Autodesk Fusion 360 part; units mm, degrees
(part 2 of 7)
  spline S12 degree 5 poles (-1.6341, -11.6319) (-1.6348, -11.637) (-1.6361, -11.6471) (-1.6376, -11.6624) (-1.639, -11.6827) (-1.6398, -11.7083) (-1.6398, -11.7339) (-1.6394, -11.7596) (-1.6387, -11.7853) (-1.6379, -11.8111) (-1.6369, -11.8368) (-1.6357, -11.8626) (-1.6342, -11.8884) (-1.6324, -11.9143) (-1.6302, -11.9401) (-1.6277, -11.966) (-1.6249, -11.9919) (-1.6219, -12.0178) (-1.6187, -12.0438) (-1.6153, -12.0697) (-1.6117, -12.0957) (-1.608, -12.1216) (-1.604, -12.1476) (-1.5998, -12.1736) (-1.5953, -12.1996) (-1.5907, -12.2256) (-1.5859, -12.2517) (-1.5809, -12.2777) (-1.5757, -12.3037) (-1.5703, -12.3298) (-1.5648, -12.3558) (-1.5591, -12.3818) (-1.5532, -12.4079) (-1.5471, -12.4339) (-1.5409, -12.46) (-1.5345, -12.4861) (-1.5279, -12.5121) (-1.5212, -12.5382) (-1.5143, -12.5642) (-1.5072, -12.5903) (-1.5, -12.6164) (-1.4927, -12.6424) (-1.4851, -12.6685) (-1.4775, -12.6945) (-1.4696, -12.7206) (-1.4617, -12.7466) (-1.4535, -12.7727) (-1.4453, -12.7987) (-1.4368, -12.8247) (-1.4283, -12.8508) (-1.4196, -12.8768) (-1.4107, -12.9028) (-1.4017, -12.9288) (-1.3926, -12.9548) (-1.3833, -12.9808) (-1.3739, -13.0068) (-1.3643, -13.0328) (-1.3546, -13.0588) (-1.3448, -13.0848) (-1.3348, -13.1107) (-1.3247, -13.1367) (-1.3144, -13.1626) (-1.3041, -13.1885) (-1.2936, -13.2145) (-1.2829, -13.2404) (-1.2721, -13.2663) (-1.2612, -13.2921) (-1.2502, -13.318) (-1.239, -13.3439) (-1.2278, -13.3697) (-1.2163, -13.3956) (-1.2071, -13.4162) (-1.2001, -13.4317) (-1.1954, -13.442) (-1.1931, -13.4472) knots 0 0 0 0 0 0 0.01428571 0.02857143 0.04285714 0.05714286 0.07142857 0.08571429 0.1 0.11428571 0.12857143 0.14285714 0.15714286 0.17142857 0.18571429 0.2 0.21428571 0.22857143 0.24285714 0.25714286 0.27142857 0.28571429 0.3 0.31428571 0.32857143 0.34285714 0.35714286 0.37142857 0.38571429 0.4 0.41428571 0.42857143 0.44285714 0.45714286 0.47142857 0.48571429 0.5 0.51428571 0.52857143 0.54285714 0.55714286 0.57142857 0.58571429 0.6 0.61428571 0.62857143 0.64285714 0.65714286 0.67142857 0.68571429 0.7 0.71428571 0.72857143 0.74285714 0.75714286 0.77142857 0.78571429 0.8 0.81428571 0.82857143 0.84285714 0.85714286 0.87142857 0.88571429 0.9 0.91428571 0.92857143 0.94285714 0.95714286 0.97142857 0.98571429 1 1 1 1 1 1
  arc A26 (-1.1931, -13.4472) -> (-0.5017, -13.4907) centre (0, 0) ccw
  spline S13 degree 5 poles (-0.5017, -13.4907) (-0.4987, -13.4858) (-0.4928, -13.4762) (-0.4839, -13.4617) (-0.4722, -13.4424) (-0.4576, -13.4182) (-0.4432, -13.3939) (-0.4288, -13.3697) (-0.4147, -13.3454) (-0.4006, -13.3211) (-0.3867, -13.2967) (-0.3729, -13.2724) (-0.3592, -13.248) (-0.3456, -13.2236) (-0.3322, -13.1991) (-0.3189, -13.1746) (-0.3058, -13.1501) (-0.2928, -13.1256) (-0.2799, -13.101) (-0.2672, -13.0765) (-0.2546, -13.0519) (-0.2421, -13.0272) (-0.2298, -13.0026) (-0.2176, -12.9779) (-0.2055, -12.9532) (-0.1936, -12.9285) (-0.1819, -12.9037) (-0.1702, -12.8789) (-0.1588, -12.8541) (-0.1474, -12.8293) (-0.1363, -12.8045) (-0.1252, -12.7796) (-0.1143, -12.7547) (-0.1036, -12.7298) (-0.093, -12.7049) (-0.0826, -12.6799) (-0.0724, -12.655) (-0.0623, -12.63) (-0.0523, -12.605) (-0.0425, -12.5799) (-0.0329, -12.5549) (-0.0235, -12.5298) (-0.0142, -12.5047) (-0.0051, -12.4796) (0.0039, -12.4545) (0.0126, -12.4293) (0.0212, -12.4042) (0.0296, -12.379) (0.0378, -12.3538) (0.0459, -12.3286) (0.0537, -12.3034) (0.0614, -12.2781) (0.0688, -12.2529) (0.076, -12.2276) (0.083, -12.2023) (0.0899, -12.177) (0.0965, -12.1517) (0.1029, -12.1264) (0.1091, -12.101) (0.1151, -12.0757) (0.1209, -12.0503) (0.1263, -12.0249) (0.1313, -11.9995) (0.136, -11.9741) (0.1404, -11.9487) (0.1447, -11.9232) (0.1487, -11.8978) (0.1526, -11.8724) (0.1562, -11.8469) (0.1594, -11.8215) (0.1619, -11.796) (0.1631, -11.7757) (0.1634, -11.7603) (0.1634, -11.7501) (0.1633, -11.745) knots -1 -1 -1 -1 -1 -1 -0.98571429 -0.97142857 -0.95714286 -0.94285714 -0.92857143 -0.91428571 -0.9 -0.88571429 -0.87142857 -0.85714286 -0.84285714 -0.82857143 -0.81428571 -0.8 -0.78571429 -0.77142857 -0.75714286 -0.74285714 -0.72857143 -0.71428571 -0.7 -0.68571429 -0.67142857 -0.65714286 -0.64285714 -0.62857143 -0.61428571 -0.6 -0.58571429 -0.57142857 -0.55714286 -0.54285714 -0.52857143 -0.51428571 -0.5 -0.48571429 -0.47142857 -0.45714286 -0.44285714 -0.42857143 -0.41428571 -0.4 -0.38571429 -0.37142857 -0.35714286 -0.34285714 -0.32857143 -0.31428571 -0.3 -0.28571429 -0.27142857 -0.25714286 -0.24285714 -0.22857143 -0.21428571 -0.2 -0.18571429 -0.17142857 -0.15714286 -0.14285714 -0.12857143 -0.11428571 -0.1 -0.08571429 -0.07142857 -0.05714286 -0.04285714 -0.02857143 -0.01428571 0 0 0 0 0 0
  line L13 (0.1633, -11.745) -> (0.1618, -11.638)
  arc A27 (0.4499, -11.3341) -> (0.1618, -11.638) centre (0.4618, -11.6338) ccw
  arc A28 (0.4499, -11.3341) -> (0.9742, -11.3011) centre (0, 0) ccw
  arc A29 (1.2981, -11.5665) -> (0.9742, -11.3011) centre (0.9999, -11.6) ccw
  line L14 (1.2981, -11.5665) -> (1.31, -11.6729)
  spline S14 degree 5 poles (1.31, -11.6729) (1.3106, -11.678) (1.3118, -11.6881) (1.3141, -11.7032) (1.3178, -11.7233) (1.3235, -11.7483) (1.3298, -11.7731) (1.3366, -11.7979) (1.3437, -11.8226) (1.3509, -11.8473) (1.3582, -11.872) (1.3658, -11.8967) (1.3737, -11.9213) (1.3819, -11.9459) (1.3904, -11.9704) (1.3992, -11.9949) (1.4084, -12.0193) (1.4177, -12.0436) (1.4273, -12.068) (1.437, -12.0922) (1.447, -12.1165) (1.4571, -12.1407) (1.4674, -12.1649) (1.478, -12.189) (1.4887, -12.2131) (1.4997, -12.2371) (1.5108, -12.2611) (1.5221, -12.2851) (1.5336, -12.309) (1.5453, -12.3329) (1.5571, -12.3568) (1.5691, -12.3806) (1.5813, -12.4043) (1.5937, -12.4281) (1.6062, -12.4518) (1.6189, -12.4754) (1.6317, -12.499) (1.6447, -12.5226) (1.6579, -12.5461) (1.6712, -12.5696) (1.6847, -12.593) (1.6983, -12.6164) (1.712, -12.6398) (1.7259, -12.6631) (1.74, -12.6864) (1.7542, -12.7097) (1.7686, -12.7329) (1.7831, -12.756) (1.7977, -12.7792) (1.8125, -12.8022) (1.8274, -12.8253) (1.8424, -12.8483) (1.8576, -12.8712) (1.8729, -12.8942) (1.8884, -12.917) (1.904, -12.9399) (1.9197, -12.9627) (1.9356, -12.9854) (1.9515, -13.0081) (1.9677, -13.0308) (1.9839, -13.0534) (2.0003, -13.076) (2.0168, -13.0985) (2.0334, -13.121) (2.0501, -13.1434) (2.067, -13.1658) (2.084, -13.1882) (2.1011, -13.2105) (2.1184, -13.2328) (2.1357, -13.255) (2.1532, -13.2772) (2.1673, -13.2949) (2.1779, -13.3082) (2.185, -13.317) (2.1886, -13.3214) knots 0 0 0 0 0 0 0.01428571 0.02857143 0.04285714 0.05714286 0.07142857 0.08571429 0.1 0.11428571 0.12857143 0.14285714 0.15714286 0.17142857 0.18571429 0.2 0.21428571 0.22857143 0.24285714 0.25714286 0.27142857 0.28571429 0.3 0.31428571 0.32857143 0.34285714 0.35714286 0.37142857 0.38571429 0.4 0.41428571 0.42857143 0.44285714 0.45714286 0.47142857 0.48571429 0.5 0.51428571 0.52857143 0.54285714 0.55714286 0.57142857 0.58571429 0.6 0.61428571 0.62857143 0.64285714 0.65714286 0.67142857 0.68571429 0.7 0.71428571 0.72857143 0.74285714 0.75714286 0.77142857 0.78571429 0.8 0.81428571 0.82857143 0.84285714 0.85714286 0.87142857 0.88571429 0.9 0.91428571 0.92857143 0.94285714 0.95714286 0.97142857 0.98571429 1 1 1 1 1 1
  arc A30 (2.1886, -13.3214) -> (2.8691, -13.1916) centre (0, 0) ccw
  spline S15 degree 5 poles (2.8691, -13.1916) (2.8707, -13.1862) (2.8741, -13.1754) (2.8791, -13.1591) (2.8857, -13.1375) (2.8937, -13.1104) (2.9017, -13.0834) (2.9095, -13.0563) (2.9172, -13.0293) (2.9248, -13.0022) (2.9323, -12.9752) (2.9396, -12.9481) (2.9467, -12.9211) (2.9538, -12.8941) (2.9607, -12.8671) (2.9675, -12.84) (2.9741, -12.813) (2.9806, -12.786) (2.987, -12.7591) (2.9932, -12.7321) (2.9993, -12.7051) (3.0053, -12.6782) (3.0111, -12.6512) (3.0167, -12.6243) (3.0223, -12.5973) (3.0276, -12.5704) (3.0329, -12.5435) (3.038, -12.5167) (3.0429, -12.4898) (3.0477, -12.4629) (3.0524, -12.4361) (3.0569, -12.4093) (3.0612, -12.3824) (3.0654, -12.3556) (3.0695, -12.3289) (3.0733, -12.3021) (3.0771, -12.2754) (3.0806, -12.2487) (3.0841, -12.222) (3.0873, -12.1953) (3.0904, -12.1686) (3.0933, -12.142) (3.0961, -12.1154) (3.0986, -12.0888) (3.101, -12.0622) (3.1033, -12.0357) (3.1053, -12.0092) (3.1072, -11.9827) (3.1089, -11.9563) (3.1105, -11.9299) (3.1118, -11.9035) (3.1129, -11.8771) (3.1138, -11.8508) (3.1145, -11.8245) (3.115, -11.7983) (3.1153, -11.7721) (3.1154, -11.7459) (3.1154, -11.7198) (3.1151, -11.6937) (3.1146, -11.6676) (3.1139, -11.6417) (3.1128, -11.6157) (3.1113, -11.5899) (3.1096, -11.5641) (3.1075, -11.5383) (3.1053, -11.5127) (3.1029, -11.487) (3.1003, -11.4614) (3.0975, -11.4359) (3.0943, -11.4105) (3.0903, -11.3852) (3.0864, -11.3652) (3.083, -11.3502) (3.0804, -11.3403) (3.0791, -11.3354) knots -1 -1 -1 -1 -1 -1 -0.98571429 -0.97142857 -0.95714286 -0.94285714 -0.92857143 -0.91428571 -0.9 -0.88571429 -0.87142857 -0.85714286 -0.84285714 -0.82857143 -0.81428571 -0.8 -0.78571429 -0.77142857 -0.75714286 -0.74285714 -0.72857143 -0.71428571 -0.7 -0.68571429 -0.67142857 -0.65714286 -0.64285714 -0.62857143 -0.61428571 -0.6 -0.58571429 -0.57142857 -0.55714286 -0.54285714 -0.52857143 -0.51428571 -0.5 -0.48571429 -0.47142857 -0.45714286 -0.44285714 -0.42857143 -0.41428571 -0.4 -0.38571429 -0.37142857 -0.35714286 -0.34285714 -0.32857143 -0.31428571 -0.3 -0.28571429 -0.27142857 -0.25714286 -0.24285714 -0.22857143 -0.21428571 -0.2 -0.18571429 -0.17142857 -0.15714286 -0.14285714 -0.12857143 -0.11428571 -0.1 -0.08571429 -0.07142857 -0.05714286 -0.04285714 -0.02857143 -0.01428571 0 0 0 0 0 0
  line L15 (3.0791, -11.3354) -> (3.051, -11.2321)
  arc A31 (3.2544, -10.8661) -> (3.051, -11.2321) centre (3.3405, -11.1535) ccw
  arc A32 (3.2544, -10.8661) -> (3.754, -10.7038) centre (0, 0) ccw
  arc A33 (4.1338, -10.8803) -> (3.754, -10.7038) centre (3.8533, -10.9869) ccw
  line L16 (4.1338, -10.8803) -> (4.1718, -10.9804)
  spline S16 degree 5 poles (4.1718, -10.9804) (4.1736, -10.9851) (4.1773, -10.9946) (4.1833, -11.0088) (4.1919, -11.0273) (4.2036, -11.05) (4.2159, -11.0725) (4.2287, -11.0948) (4.2416, -11.117) (4.2547, -11.1392) (4.268, -11.1613) (4.2815, -11.1833) (4.2952, -11.2052) (4.3093, -11.227) (4.3236, -11.2486) (4.3383, -11.2701) (4.3532, -11.2914) (4.3683, -11.3127) (4.3836, -11.3339) (4.3991, -11.355) (4.4148, -11.376) (4.4306, -11.3969) (4.4466, -11.4178) (4.4628, -11.4385) (4.4792, -11.4592) (4.4958, -11.4797) (4.5126, -11.5002) (4.5295, -11.5206) (4.5466, -11.5409) (4.5638, -11.5612) (4.5812, -11.5813) (4.5988, -11.6014) (4.6165, -11.6214) (4.6343, -11.6413) (4.6524, -11.6611) (4.6705, -11.6809) (4.6888, -11.7005) (4.7073, -11.7201) (4.7259, -11.7396) (4.7446, -11.7591) (4.7635, -11.7784) (4.7825, -11.7977) (4.8016, -11.8169) (4.8209, -11.8361) (4.8403, -11.8551) (4.8599, -11.8741) (4.8795, -11.893) (4.8993, -11.9119) (4.9193, -11.9306) (4.9393, -11.9493) (4.9595, -11.9679) (4.9798, -11.9864) (5.0002, -12.0049) (5.0207, -12.0233) (5.0414, -12.0416) (5.0622, -12.0598) (5.0831, -12.078) (5.1041, -12.0961) (5.1252, -12.1141) (5.1465, -12.1321) (5.1678, -12.1499) (5.1893, -12.1677) (5.2109, -12.1854) (5.2326, -12.2031) (5.2544, -12.2207) (5.2763, -12.2382) (5.2983, -12.2556) (5.3204, -12.273) (5.3427, -12.2902) (5.365, -12.3074) (5.3875, -12.3246) (5.4055, -12.3382) (5.4191, -12.3484) (5.4282, -12.3552) (5.4327, -12.3586) knots 0 0 0 0 0 0 0.01428571 0.02857143 0.04285714 0.05714286 0.07142857 0.08571429 0.1 0.11428571 0.12857143 0.14285714 0.15714286 0.17142857 0.18571429 0.2 0.21428571 0.22857143 0.24285714 0.25714286 0.27142857 0.28571429 0.3 0.31428571 0.32857143 0.34285714 0.35714286 0.37142857 0.38571429 0.4 0.41428571 0.42857143 0.44285714 0.45714286 0.47142857 0.48571429 0.5 0.51428571 0.52857143 0.54285714 0.55714286 0.57142857 0.58571429 0.6 0.61428571 0.62857143 0.64285714 0.65714286 0.67142857 0.68571429 0.7 0.71428571 0.72857143 0.74285714 0.75714286 0.77142857 0.78571429 0.8 0.81428571 0.82857143 0.84285714 0.85714286 0.87142857 0.88571429 0.9 0.91428571 0.92857143 0.94285714 0.95714286 0.97142857 0.98571429 1 1 1 1 1 1
  arc A34 (5.4327, -12.3586) -> (6.0595, -12.0637) centre (0, 0) ccw
  spline S17 degree 5 poles (6.0595, -12.0637) (6.0598, -12.058) (6.0604, -12.0467) (6.0612, -12.0297) (6.0622, -12.0071) (6.0633, -11.9789) (6.0642, -11.9507) (6.0651, -11.9225) (6.0658, -11.8944) (6.0664, -11.8663) (6.0669, -11.8383) (6.0673, -11.8103) (6.0675, -11.7823) (6.0676, -11.7544) (6.0676, -11.7265) (6.0674, -11.6987) (6.0671, -11.6709) (6.0667, -11.6431) (6.0662, -11.6154) (6.0655, -11.5877) (6.0647, -11.5601) (6.0638, -11.5325) (6.0627, -11.5049) (6.0615, -11.4774) (6.0601, -11.45) (6.0587, -11.4226) (6.057, -11.3952) (6.0553, -11.3679) (6.0534, -11.3406) (6.0514, -11.3134) (6.0492, -11.2863) (6.0469, -11.2592) (6.0444, -11.2321) (6.0418, -11.2051) (6.0391, -11.1782) (6.0362, -11.1513) (6.0332, -11.1245) (6.03, -11.0977) (6.0266, -11.071) (6.0232, -11.0444) (6.0195, -11.0178) (6.0157, -10.9913) (6.0118, -10.9648) (6.0077, -10.9384) (6.0034, -10.9121) (5.9989, -10.8858) (5.9943, -10.8597) (5.9896, -10.8335) (5.9847, -10.8075) (5.9796, -10.7815) (5.9743, -10.7556) (5.9688, -10.7298) (5.9632, -10.7041) (5.9573, -10.6785) (5.9513, -10.653) (5.9451, -10.6275) (5.9387, -10.6021) (5.9321, -10.5768) (5.9254, -10.5516) (5.9184, -10.5265) (5.9112, -10.5015) (5.9037, -10.4767) (5.8959, -10.452) (5.8878, -10.4274) (5.8794, -10.403) (5.8708, -10.3787) (5.8621, -10.3545) (5.8533, -10.3303) (5.8442, -10.3063) (5.8347, -10.2825) (5.8246, -10.259) (5.8159, -10.2405) (5.8088, -10.2269) (5.8038, -10.218) (5.8013, -10.2136) knots -1 -1 -1 -1 -1 -1 -0.98571429 -0.97142857 -0.95714286 -0.94285714 -0.92857143 -0.91428571 -0.9 -0.88571429 -0.87142857 -0.85714286 -0.84285714 -0.82857143 -0.81428571 -0.8 -0.78571429 -0.77142857 -0.75714286 -0.74285714 -0.72857143 -0.71428571 -0.7 -0.68571429 -0.67142857 -0.65714286 -0.64285714 -0.62857143 -0.61428571 -0.6 -0.58571429 -0.57142857 -0.55714286 -0.54285714 -0.52857143 -0.51428571 -0.5 -0.48571429 -0.47142857 -0.45714286 -0.44285714 -0.42857143 -0.41428571 -0.4 -0.38571429 -0.37142857 -0.35714286 -0.34285714 -0.32857143 -0.31428571 -0.3 -0.28571429 -0.27142857 -0.25714286 -0.24285714 -0.22857143 -0.21428571 -0.2 -0.18571429 -0.17142857 -0.15714286 -0.14285714 -0.12857143 -0.11428571 -0.1 -0.08571429 -0.07142857 -0.05714286 -0.04285714 -0.02857143 -0.01428571 0 0 0 0 0 0
  line L17 (5.8013, -10.2136) -> (5.7485, -10.1205)
  arc A35 (5.8545, -9.7154) -> (5.7485, -10.1205) centre (6.0093, -9.9723) ccw
  arc A36 (5.8545, -9.7154) -> (6.298, -9.4339) centre (0, 0) ccw
  arc A37 (6.7097, -9.5105) -> (6.298, -9.4339) centre (6.4646, -9.6834) ccw
  line L18 (6.7097, -9.5105) -> (6.7714, -9.5979)
  spline S18 degree 5 poles (6.7714, -9.5979) (6.7744, -9.6021) (6.7804, -9.6104) (6.7896, -9.6225) (6.8026, -9.6383) (6.8196, -9.6575) (6.8371, -9.6762) (6.855, -9.6946) (6.8731, -9.7129) (6.8913, -9.7311) (6.9096, -9.7492) (6.9281, -9.7672) (6.9469, -9.785) (6.9659, -9.8026) (6.9852, -9.8199) (7.0047, -9.8371) (7.0245, -9.8541) (7.0444, -9.8709) (7.0645, -9.8876) (7.0848, -9.9042) (7.1052, -9.9207) (7.1257, -9.937) (7.1464, -9.9532) (7.1672, -9.9693) (7.1883, -9.9852) (7.2094, -10.001) (7.2308, -10.0167) (7.2522, -10.0322) (7.2738, -10.0477) (7.2956, -10.063) (7.3174, -10.0782) (7.3394, -10.0932) (7.3616, -10.1082) (7.3838, -10.123) (7.4062, -10.1378) (7.4287, -10.1524) (7.4513, -10.1669) (7.4741, -10.1813) (7.4969, -10.1955) (7.5199, -10.2097) (7.543, -10.2238) (7.5662, -10.2377) (7.5895, -10.2516) (7.613, -10.2653) (7.6365, -10.2789) (7.6602, -10.2925) (7.6839, -10.3059) (7.7078, -10.3192) (7.7317, -10.3324) (7.7558, -10.3455) (7.78, -10.3585) (7.8042, -10.3714) (7.8286, -10.3842) (7.8531, -10.3969) (7.8776, -10.4095) (7.9023, -10.422) (7.9271, -10.4344) (7.9519, -10.4467) (7.9768, -10.4589) (8.0019, -10.471) (8.027, -10.483) (8.0522, -10.4949) (8.0776, -10.5067) (8.103, -10.5184) (8.1284, -10.53) (8.154, -10.5415) (8.1797, -10.5529) (8.2054, -10.5642) (8.2313, -10.5754) (8.2572, -10.5866) (8.2832, -10.5976) (8.3041, -10.6063) (8.3198, -10.6128) (8.3303, -10.6171) (8.3355, -10.6193) knots 0 0 0 0 0 0 0.01428571 0.02857143 0.04285714 0.05714286 0.07142857 0.08571429 0.1 0.11428571 0.12857143 0.14285714 0.15714286 0.17142857 0.18571429 0.2 0.21428571 0.22857143 0.24285714 0.25714286 0.27142857 0.28571429 0.3 0.31428571 0.32857143 0.34285714 0.35714286 0.37142857 0.38571429 0.4 0.41428571 0.42857143 0.44285714 0.45714286 0.47142857 0.48571429 0.5 0.51428571 0.52857143 0.54285714 0.55714286 0.57142857 0.58571429 0.6 0.61428571 0.62857143 0.64285714 0.65714286 0.67142857 0.68571429 0.7 0.71428571 0.72857143 0.74285714 0.75714286 0.77142857 0.78571429 0.8 0.81428571 0.82857143 0.84285714 0.85714286 0.87142857 0.88571429 0.9 0.91428571 0.92857143 0.94285714 0.95714286 0.97142857 0.98571429 1 1 1 1 1 1
  arc A38 (8.3355, -10.6193) -> (8.8693, -10.1777) centre (0, 0) ccw
  spline S19 degree 5 poles (8.8693, -10.1777) (8.8681, -10.1722) (8.8659, -10.1611) (8.8624, -10.1444) (8.8577, -10.1223) (8.8518, -10.0947) (8.8457, -10.0671) (8.8396, -10.0396) (8.8333, -10.0122) (8.8269, -9.9849) (8.8204, -9.9576) (8.8138, -9.9304) (8.807, -9.9032) (8.8002, -9.8762) (8.7932, -9.8492) (8.7862, -9.8222) (8.779, -9.7954) (8.7717, -9.7686) (8.7642, -9.7419) (8.7567, -9.7152) (8.749, -9.6887) (8.7413, -9.6622) (8.7334, -9.6357) (8.7254, -9.6094) (8.7172, -9.5832) (8.709, -9.557) (8.7006, -9.5309) (8.6921, -9.5049) (8.6835, -9.4789) (8.6748, -9.4531) (8.6659, -9.4273) (8.657, -9.4017) (8.6479, -9.3761) (8.6386, -9.3506) (8.6293, -9.3252) (8.6198, -9.2998) (8.6102, -9.2746) (8.6004, -9.2495) (8.5906, -9.2244) (8.5806, -9.1995) (8.5704, -9.1746) (8.5601, -9.1499) (8.5497, -9.1253) (8.5392, -9.1007) (8.5285, -9.0763) (8.5177, -9.052) (8.5067, -9.0277) (8.4956, -9.0036) (8.4844, -8.9796) (8.473, -8.9557) (8.4614, -8.932) (8.4497, -8.9083) (8.4378, -8.8848) (8.4258, -8.8615) (8.4136, -8.8383) (8.4012, -8.8151) (8.3887, -8.7922) (8.3761, -8.7693) (8.3633, -8.7465) (8.3503, -8.724) (8.3371, -8.7015) (8.3237, -8.6793) (8.31, -8.6574) (8.296, -8.6356) (8.2818, -8.6141) (8.2675, -8.5926) (8.253, -8.5713) (8.2384, -8.5501) (8.2237, -8.5291) (8.2086, -8.5084) (8.1929, -8.4881) (8.1799, -8.4725) (8.1696, -8.4611) (8.1626, -8.4536) (8.1591, -8.45) knots -1 -1 -1 -1 -1 -1 -0.98571429 -0.97142857 -0.95714286 -0.94285714 -0.92857143 -0.91428571 -0.9 -0.88571429 -0.87142857 -0.85714286 -0.84285714 -0.82857143 -0.81428571 -0.8 -0.78571429 -0.77142857 -0.75714286 -0.74285714 -0.72857143 -0.71428571 -0.7 -0.68571429 -0.67142857 -0.65714286 -0.64285714 -0.62857143 -0.61428571 -0.6 -0.58571429 -0.57142857 -0.55714286 -0.54285714 -0.52857143 -0.51428571 -0.5 -0.48571429 -0.47142857 -0.45714286 -0.44285714 -0.42857143 -0.41428571 -0.4 -0.38571429 -0.37142857 -0.35714286 -0.34285714 -0.32857143 -0.31428571 -0.3 -0.28571429 -0.27142857 -0.25714286 -0.24285714 -0.22857143 -0.21428571 -0.2 -0.18571429 -0.17142857 -0.15714286 -0.14285714 -0.12857143 -0.11428571 -0.1 -0.08571429 -0.07142857 -0.05714286 -0.04285714 -0.02857143 -0.01428571 0 0 0 0 0 0
  line L19 (8.1591, -8.45) -> (8.0847, -8.373)
  arc A39 (8.0867, -7.9542) -> (8.0847, -8.373) centre (8.3005, -8.1646) ccw
  arc A40 (8.0867, -7.9542) -> (8.4463, -7.5713) centre (0, 0) ccw
  arc A41 (8.8641, -7.543) -> (8.4463, -7.5713) centre (8.6697, -7.7715) ccw
  line L20 (8.8641, -7.543) -> (8.9456, -7.6124)
  spline S20 degree 5 poles (8.9456, -7.6124) (8.9495, -7.6157) (8.9573, -7.6222) (8.9694, -7.6317) (8.9858, -7.6438) (9.007, -7.6581) (9.0287, -7.6719) (9.0506, -7.6853) (9.0726, -7.6985) (9.0948, -7.7116) (9.1171, -7.7246) (9.1395, -7.7374) (9.1621, -7.75) (9.1849, -7.7623) (9.2079, -7.7743) (9.2311, -7.786) (9.2544, -7.7976) (9.2779, -7.8089) (9.3015, -7.8201) (9.3253, -7.8311) (9.3491, -7.842) (9.3731, -7.8527) (9.3971, -7.8633) (9.4213, -7.8737) (9.4457, -7.8839) (9.4701, -7.8939) (9.4947, -7.9038) (9.5193, -7.9135) (9.5441, -7.9231) (9.5689, -7.9325) (9.5939, -7.9418) (9.6189, -7.9509) (9.6441, -7.9599) (9.6693, -7.9687) (9.6947, -7.9774) (9.7201, -7.986) (9.7456, -7.9944) (9.7712, -8.0027) (9.7969, -8.0108) (9.8227, -8.0188) (9.8486, -8.0267) (9.8745, -8.0344) (9.9006, -8.0421) (9.9267, -8.0495) (9.9529, -8.0569) (9.9791, -8.0641) (10.0055, -8.0712) (10.0319, -8.0782) (10.0584, -8.085) (10.085, -8.0917) (10.1116, -8.0983) (10.1383, -8.1048) (10.1651, -8.1111) (10.192, -8.1173) (10.2189, -8.1234) (10.2459, -8.1294) (10.2729, -8.1352) (10.3001, -8.141) (10.3273, -8.1466) (10.3545, -8.1521) (10.3819, -8.1574) (10.4092, -8.1627) (10.4367, -8.1678) (10.4642, -8.1728) (10.4918, -8.1777) (10.5194, -8.1825) (10.5471, -8.1872) (10.5749, -8.1917) (10.6027, -8.1962) (10.6306, -8.2005) (10.6585, -8.2047) (10.6809, -8.2079) (10.6977, -8.2103) (10.7089, -8.2119) (10.7145, -8.2127) knots 0 0 0 0 0 0 0.01428571 0.02857143 0.04285714 0.05714286 0.07142857 0.08571429 0.1 0.11428571 0.12857143 0.14285714 0.15714286 0.17142857 0.18571429 0.2 0.21428571 0.22857143 0.24285714 0.25714286 0.27142857 0.28571429 0.3 0.31428571 0.32857143 0.34285714 0.35714286 0.37142857 0.38571429 0.4 0.41428571 0.42857143 0.44285714 0.45714286 0.47142857 0.48571429 0.5 0.51428571 0.52857143 0.54285714 0.55714286 0.57142857 0.58571429 0.6 0.61428571 0.62857143 0.64285714 0.65714286 0.67142857 0.68571429 0.7 0.71428571 0.72857143 0.74285714 0.75714286 0.77142857 0.78571429 0.8 0.81428571 0.82857143 0.84285714 0.85714286 0.87142857 0.88571429 0.9 0.91428571 0.92857143 0.94285714 0.95714286 0.97142857 0.98571429 1 1 1 1 1 1
  arc A42 (10.7145, -8.2127) -> (11.1217, -7.6523) centre (0, 0) ccw
  spline S21 degree 5 poles (11.1217, -7.6523) (11.1192, -7.6472) (11.1143, -7.637) (11.1068, -7.6217) (11.0968, -7.6014) (11.0841, -7.5762) (11.0714, -7.551) (11.0586, -7.5259) (11.0457, -7.5009) (11.0327, -7.476) (11.0196, -7.4512) (11.0065, -7.4265) (10.9932, -7.4019) (10.9798, -7.3774) (10.9664, -7.3529) (10.9528, -7.3286) (10.9392, -7.3044) (10.9254, -7.2803) (10.9116, -7.2562) (10.8977, -7.2323) (10.8836, -7.2085) (10.8695, -7.1847) (10.8553, -7.1611) (10.841, -7.1376) (10.8266, -7.1142) (10.8121, -7.0909) (10.7975, -7.0677) (10.7828, -7.0446) (10.768, -7.0216) (10.7531, -6.9988) (10.7382, -6.976) (10.7231, -6.9534) (10.7079, -6.9309) (10.6926, -6.9085) (10.6772, -6.8862) (10.6617, -6.864) (10.6462, -6.842) (10.6305, -6.82) (10.6147, -6.7982) (10.5988, -6.7766) (10.5828, -6.755) (10.5667, -6.7336) (10.5505, -6.7123) (10.5342, -6.6912) (10.5177, -6.6702) (10.5012, -6.6493) (10.4846, -6.6286) (10.4678, -6.608) (10.4509, -6.5875) (10.434, -6.5672) (10.4169, -6.5471) (10.3997, -6.5271) (10.3823, -6.5073) (10.3648, -6.4877) (10.3472, -6.4682) (10.3295, -6.4489) (10.3117, -6.4297) (10.2938, -6.4107) (10.2757, -6.3919) (10.2575, -6.3732) (10.2392, -6.3548) (10.2206, -6.3367) (10.2019, -6.3188) (10.1829, -6.3012) (10.1638, -6.2838) (10.1446, -6.2666) (10.1253, -6.2496) (10.1059, -6.2327) (10.0864, -6.216) (10.0666, -6.1997) (10.0465, -6.184) (10.0299, -6.172) (10.0171, -6.1635) (10.0085, -6.1581) (10.0042, -6.1554) knots -1 -1 -1 -1 -1 -1 -0.98571429 -0.97142857 -0.95714286 -0.94285714 -0.92857143 -0.91428571 -0.9 -0.88571429 -0.87142857 -0.85714286 -0.84285714 -0.82857143 -0.81428571 -0.8 -0.78571429 -0.77142857 -0.75714286 -0.74285714 -0.72857143 -0.71428571 -0.7 -0.68571429 -0.67142857 -0.65714286 -0.64285714 -0.62857143 -0.61428571 -0.6 -0.58571429 -0.57142857 -0.55714286 -0.54285714 -0.52857143 -0.51428571 -0.5 -0.48571429 -0.47142857 -0.45714286 -0.44285714 -0.42857143 -0.41428571 -0.4 -0.38571429 -0.37142857 -0.35714286 -0.34285714 -0.32857143 -0.31428571 -0.3 -0.28571429 -0.27142857 -0.25714286 -0.24285714 -0.22857143 -0.21428571 -0.2 -0.18571429 -0.17142857 -0.15714286 -0.14285714 -0.12857143 -0.11428571 -0.1 -0.08571429 -0.07142857 -0.05714286 -0.04285714 -0.02857143 -0.01428571 0 0 0 0 0 0
  line L21 (10.0042, -6.1554) -> (9.913, -6.0993)
  arc A43 (9.8107, -5.6932) -> (9.913, -6.0993) centre (10.0702, -5.8438) ccw
  arc A44 (9.8107, -5.6932) -> (10.0638, -5.2329) centre (0, 0) ccw
  arc A45 (10.4615, -5.1017) -> (10.0638, -5.2329) centre (10.33, -5.3713) ccw
  line L22 (10.4615, -5.1017) -> (10.5577, -5.1486)
  spline S22 degree 5 poles (10.5577, -5.1486) (10.5623, -5.1508) (10.5715, -5.1552) (10.5855, -5.1614) (10.6045, -5.169) (10.6285, -5.1776) (10.6529, -5.1855) (10.6775, -5.1931) (10.7021, -5.2004) (10.7269, -5.2076) (10.7517, -5.2146) (10.7766, -5.2214) (10.8016, -5.228) (10.8267, -5.2342) (10.852, -5.2401) (10.8774, -5.2458) (10.9029, -5.2511) (10.9284, -5.2563) (10.9541, -5.2612) (10.9798, -5.266) (11.0056, -5.2706) (11.0315, -5.2751) (11.0574, -5.2793) (11.0834, -5.2833) (11.1095, -5.2872) (11.1357, -5.2908) (11.1619, -5.2942) (11.1883, -5.2975) (11.2146, -5.3006) (11.241, -5.3036) (11.2675, -5.3064) (11.2941, -5.309) (11.3206, -5.3114) (11.3473, -5.3137) (11.374, -5.3158) (11.4008, -5.3178) (11.4276, -5.3196) (11.4544, -5.3212) (11.4814, -5.3227) (11.5083, -5.3241) (11.5353, -5.3253) (11.5624, -5.3263) (11.5895, -5.3272) (11.6166, -5.328) (11.6438, -5.3286) (11.6711, -5.3291) (11.6984, -5.3294) (11.7257, -5.3295) (11.7531, -5.3296) (11.7805, -5.3295) (11.8079, -5.3292) (11.8354, -5.3288) (11.8629, -5.3283) (11.8905, -5.3277) (11.9181, -5.3269) (11.9457, -5.3259) (11.9734, -5.3249) (12.0011, -5.3237) (12.0288, -5.3224) (12.0566, -5.3209) (12.0844, -5.3193) (12.1122, -5.3176) (12.1401, -5.3157) (12.168, -5.3137) (12.1959, -5.3116) (12.2238, -5.3094) (12.2518, -5.307) (12.2798, -5.3045) (12.3079, -5.3019) (12.336, -5.2991) (12.3641, -5.2963) (12.3866, -5.2939) (12.4034, -5.292) (12.4147, -5.2907) (12.4203, -5.2901) knots 0 0 0 0 0 0 0.01428571 0.02857143 0.04285714 0.05714286 0.07142857 0.08571429 0.1 0.11428571 0.12857143 0.14285714 0.15714286 0.17142857 0.18571429 0.2 0.21428571 0.22857143 0.24285714 0.25714286 0.27142857 0.28571429 0.3 0.31428571 0.32857143 0.34285714 0.35714286 0.37142857 0.38571429 0.4 0.41428571 0.42857143 0.44285714 0.45714286 0.47142857 0.48571429 0.5 0.51428571 0.52857143 0.54285714 0.55714286 0.57142857 0.58571429 0.6 0.61428571 0.62857143 0.64285714 0.65714286 0.67142857 0.68571429 0.7 0.71428571 0.72857143 0.74285714 0.75714286 0.77142857 0.78571429 0.8 0.81428571 0.82857143 0.84285714 0.85714286 0.87142857 0.88571429 0.9 0.91428571 0.92857143 0.94285714 0.95714286 0.97142857 0.98571429 1 1 1 1 1 1
  arc A46 (12.4203, -5.2901) -> (12.6754, -4.646) centre (0, 0) ccw
  spline S23 degree 5 poles (12.6754, -4.646) (12.6717, -4.6417) (12.6643, -4.633) (12.6533, -4.6201) (12.6385, -4.603) (12.62, -4.5816) (12.6015, -4.5604) (12.5828, -4.5393) (12.5641, -4.5183) (12.5453, -4.4974) (12.5265, -4.4767) (12.5076, -4.456) (12.4886, -4.4355) (12.4695, -4.415) (12.4504, -4.3947) (12.4313, -4.3745) (12.412, -4.3544) (12.3927, -4.3345) (12.3733, -4.3147) (12.3539, -4.2949) (12.3344, -4.2753) (12.3148, -4.2559) (12.2952, -4.2365) (12.2755, -4.2173) (12.2557, -4.1982) (12.2359, -4.1793) (12.216, -4.1604) (12.196, -4.1417) (12.1759, -4.1231) (12.1558, -4.1047) (12.1357, -4.0864) (12.1154, -4.0682) (12.0951, -4.0502) (12.0748, -4.0323) (12.0543, -4.0145) (12.0338, -3.9969) (12.0132, -3.9794) (11.9926, -3.9621) (11.9719, -3.9449) (11.9511, -3.9279) (11.9302, -3.911) (11.9093, -3.8942) (11.8883, -3.8777) (11.8672, -3.8612) (11.8461, -3.845) (11.8249, -3.8289) (11.8036, -3.8129) (11.7823, -3.7972) (11.7609, -3.7815) (11.7394, -3.7661) (11.7178, -3.7508) (11.6962, -3.7358) (11.6744, -3.7209) (11.6526, -3.7062) (11.6307, -3.6917) (11.6088, -3.6774) (11.5868, -3.6633) (11.5646, -3.6494) (11.5425, -3.6356) (11.5202, -3.6221) (11.4979, -3.6088) (11.4754, -3.5958) (11.4528, -3.5832) (11.4301, -3.5708) (11.4073, -3.5588) (11.3844, -3.5469) (11.3614, -3.5352) (11.3384, -3.5237) (11.3154, -3.5123) (11.2922, -3.5015) (11.2687, -3.4912) (11.2497, -3.4838) (11.2353, -3.4787) (11.2255, -3.4756) (11.2206, -3.4741) knots -1 -1 -1 -1 -1 -1 -0.98571429 -0.97142857 -0.95714286 -0.94285714 -0.92857143 -0.91428571 -0.9 -0.88571429 -0.87142857 -0.85714286 -0.84285714 -0.82857143 -0.81428571 -0.8 -0.78571429 -0.77142857 -0.75714286 -0.74285714 -0.72857143 -0.71428571 -0.7 -0.68571429 -0.67142857 -0.65714286 -0.64285714 -0.62857143 -0.61428571 -0.6 -0.58571429 -0.57142857 -0.55714286 -0.54285714 -0.52857143 -0.51428571 -0.5 -0.48571429 -0.47142857 -0.45714286 -0.44285714 -0.42857143 -0.41428571 -0.4 -0.38571429 -0.37142857 -0.35714286 -0.34285714 -0.32857143 -0.31428571 -0.3 -0.28571429 -0.27142857 -0.25714286 -0.24285714 -0.22857143 -0.21428571 -0.2 -0.18571429 -0.17142857 -0.15714286 -0.14285714 -0.12857143 -0.11428571 -0.1 -0.08571429 -0.07142857 -0.05714286 -0.04285714 -0.02857143 -0.01428571 0 0 0 0 0 0
  line L23 (11.2206, -3.4741) -> (11.1184, -3.4424)
  arc A47 (10.9184, -3.0745) -> (11.1184, -3.4424) centre (11.2071, -3.1559) ccw
  arc A48 (10.9184, -3.0745) -> (11.049, -2.5657) centre (0, 0) ccw
  arc A49 (11.4015, -2.3397) -> (11.049, -2.5657) centre (11.3412, -2.6336) ccw
  line L24 (11.4015, -2.3397) -> (11.5064, -2.3612)
  spline S24 degree 5 poles (11.5064, -2.3612) (11.5114, -2.3623) (11.5214, -2.3642) (11.5365, -2.3667) (11.5568, -2.3694) (11.5822, -2.3717) (11.6078, -2.3733) (11.6335, -2.3745) (11.6592, -2.3755) (11.6849, -2.3763) (11.7107, -2.3769) (11.7365, -2.3773) (11.7624, -2.3775) (11.7883, -2.3773) (11.8142, -2.3767) (11.8402, -2.3759) (11.8662, -2.3747) (11.8923, -2.3733) (11.9184, -2.3718) (11.9445, -2.37) (11.9706, -2.3681) (11.9968, -2.3659) (12.0229, -2.3636) (12.0491, -2.361) (12.0754, -2.3582) (12.1016, -2.3552) (12.1279, -2.352) (12.1542, -2.3487) (12.1805, -2.3451) (12.2068, -2.3414) (12.2332, -2.3375) (12.2595, -2.3335) (12.2859, -2.3292) (12.3123, -2.3248) (12.3387, -2.3202) (12.3651, -2.3155) (12.3915, -2.3105) (12.4179, -2.3055) (12.4444, -2.3002) (12.4708, -2.2948) (12.4973, -2.2893) (12.5237, -2.2835) (12.5502, -2.2777) (12.5767, -2.2717) (12.6032, -2.2655) (12.6297, -2.2592) (12.6562, -2.2527) (12.6827, -2.2461) (12.7092, -2.2393) (12.7357, -2.2324) (12.7623, -2.2253) (12.7888, -2.2181) (12.8153, -2.2107) (12.8418, -2.2033) (12.8684, -2.1956) (12.8949, -2.1879) (12.9214, -2.1799) (12.948, -2.1719) (12.9745, -2.1637) (13.001, -2.1554) (13.0276, -2.1469) (13.0541, -2.1383) (13.0806, -2.1296) (13.1072, -2.1207) (13.1337, -2.1118) (13.1602, -2.1026) (13.1867, -2.0934) (13.2132, -2.084) (13.2397, -2.0745) (13.2662, -2.0648) (13.2927, -2.055) (13.3139, -2.0471) (13.3298, -2.0411) (13.3404, -2.0371) (13.3457, -2.0351) knots 0 0 0 0 0 0 0.01428571 0.02857143 0.04285714 0.05714286 0.07142857 0.08571429 0.1 0.11428571 0.12857143 0.14285714 0.15714286 0.17142857 0.18571429 0.2 0.21428571 0.22857143 0.24285714 0.25714286 0.27142857 0.28571429 0.3 0.31428571 0.32857143 0.34285714 0.35714286 0.37142857 0.38571429 0.4 0.41428571 0.42857143 0.44285714 0.45714286 0.47142857 0.48571429 0.5 0.51428571 0.52857143 0.54285714 0.55714286 0.57142857 0.58571429 0.6 0.61428571 0.62857143 0.64285714 0.65714286 0.67142857 0.68571429 0.7 0.71428571 0.72857143 0.74285714 0.75714286 0.77142857 0.78571429 0.8 0.81428571 0.82857143 0.84285714 0.85714286 0.87142857 0.88571429 0.9 0.91428571 0.92857143 0.94285714 0.95714286 0.97142857 0.98571429 1 1 1 1 1 1
  arc A50 (13.3457, -2.0351) -> (13.4326, -1.3478) centre (0, 0) ccw
  spline S25 degree 5 poles (13.4326, -1.3478) (13.4279, -1.3445) (13.4187, -1.338) (13.4048, -1.3282) (13.3862, -1.3153) (13.363, -1.2992) (13.3397, -1.2833) (13.3164, -1.2675) (13.293, -1.2518) (13.2697, -1.2362) (13.2462, -1.2208) (13.2228, -1.2055) (13.1993, -1.1903) (13.1758, -1.1753) (13.1522, -1.1604) (13.1286, -1.1456) (13.105, -1.1309) (13.0813, -1.1164) (13.0576, -1.102) (13.0339, -1.0877) (13.0101, -1.0736) (12.9863, -1.0596) (12.9625, -1.0457) (12.9386, -1.032) (12.9147, -1.0185) (12.8908, -1.005) (12.8668, -0.9917) (12.8428, -0.9786) (12.8188, -0.9656) (12.7947, -0.9527) (12.7706, -0.94) (12.7465, -0.9274) (12.7224, -0.915) (12.6982, -0.9027) (12.674, -0.8906) (12.6497, -0.8786) (12.6254, -0.8668) (12.6011, -0.8552) (12.5768, -0.8437) (12.5524, -0.8323) (12.528, -0.8212) (12.5036, -0.8102) (12.4792, -0.7993) (12.4547, -0.7887) (12.4302, -0.7782) (12.4056, -0.7679) (12.381, -0.7577) (12.3564, -0.7477) (12.3318, -0.7379) (12.3072, -0.7283) (12.2825, -0.7189) (12.2578, -0.7097) (12.233, -0.7007) (12.2082, -0.6919) (12.1834, -0.6833) (12.1586, -0.6749) (12.1338, -0.6667) (12.1089, -0.6587) (12.084, -0.6509) (12.0591, -0.6433) (12.0341, -0.636) (12.0091, -0.629) (11.9841, -0.6224) (11.959, -0.6161) (11.9339, -0.6101) (11.9088, -0.6043) (11.8837, -0.5987) (11.8585, -0.5932) (11.8334, -0.588) (11.8082, -0.5832) (11.7829, -0.5791) (11.7627, -0.5767) (11.7474, -0.5754) (11.7372, -0.5747) (11.7321, -0.5745) knots -1 -1 -1 -1 -1 -1 -0.98571429 -0.97142857 -0.95714286 -0.94285714 -0.92857143 -0.91428571 -0.9 -0.88571429 -0.87142857 -0.85714286 -0.84285714 -0.82857143 -0.81428571 -0.8 -0.78571429 -0.77142857 -0.75714286 -0.74285714 -0.72857143 -0.71428571 -0.7 -0.68571429 -0.67142857 -0.65714286 -0.64285714 -0.62857143 -0.61428571 -0.6 -0.58571429 -0.57142857 -0.55714286 -0.54285714 -0.52857143 -0.51428571 -0.5 -0.48571429 -0.47142857 -0.45714286 -0.44285714 -0.42857143 -0.41428571 -0.4 -0.38571429 -0.37142857 -0.35714286 -0.34285714 -0.32857143 -0.31428571 -0.3 -0.28571429 -0.27142857 -0.25714286 -0.24285714 -0.22857143 -0.21428571 -0.2 -0.18571429 -0.17142857 -0.15714286 -0.14285714 -0.12857143 -0.11428571 -0.1 -0.08571429 -0.07142857 -0.05714286 -0.04285714 -0.02857143 -0.01428571 0 0 0 0 0 0
  line L25 (11.7321, -0.5745) -> (11.6252, -0.5692)
  arc A51 (11.34, -0.2627) -> (11.6252, -0.5692) centre (11.6399, -0.2696) ccw
  arc A52 (11.34, -0.2627) -> (11.34, 0.2627) centre (0, 0) ccw
  arc A53 (11.6252, 0.5692) -> (11.34, 0.2627) centre (11.6399, 0.2696) ccw
  line L26 (11.6252, 0.5692) -> (11.7321, 0.5745)
  spline S26 degree 5 poles (11.7321, 0.5745) (11.7372, 0.5747) (11.7474, 0.5754) (11.7627, 0.5767) (11.7829, 0.5791) (11.8082, 0.5832) (11.8334, 0.588) (11.8585, 0.5932) (11.8837, 0.5987) (11.9088, 0.6043) (11.9339, 0.6101) (11.959, 0.6161) (11.9841, 0.6224) (12.0091, 0.629) (12.0341, 0.636) (12.0591, 0.6433) (12.084, 0.6509) (12.1089, 0.6587) (12.1338, 0.6667) (12.1586, 0.6749) (12.1834, 0.6833) (12.2082, 0.6919) (12.233, 0.7007) (12.2578, 0.7097) (12.2825, 0.7189) (12.3072, 0.7283) (12.3318, 0.7379) (12.3564, 0.7477) (12.381, 0.7577) (12.4056, 0.7679) (12.4302, 0.7782) (12.4547, 0.7887) (12.4792, 0.7993) (12.5036, 0.8102) (12.528, 0.8212) (12.5524, 0.8323) (12.5768, 0.8437) (12.6011, 0.8552) (12.6254, 0.8668) (12.6497, 0.8786) (12.674, 0.8906) (12.6982, 0.9027) (12.7224, 0.915) (12.7465, 0.9274) (12.7706, 0.94) (12.7947, 0.9527) (12.8188, 0.9656) (12.8428, 0.9786) (12.8668, 0.9917) (12.8908, 1.005) (12.9147, 1.0185) (12.9386, 1.032) (12.9625, 1.0457) (12.9863, 1.0596) (13.0101, 1.0736) (13.0339, 1.0877) (13.0576, 1.102) (13.0813, 1.1164) (13.105, 1.1309) (13.1286, 1.1456) (13.1522, 1.1604) (13.1758, 1.1753) (13.1993, 1.1903) (13.2228, 1.2055) (13.2462, 1.2208) (13.2697, 1.2362) (13.293, 1.2518) (13.3164, 1.2675) (13.3397, 1.2833) (13.363, 1.2992) (13.3862, 1.3153) (13.4048, 1.3282) (13.4187, 1.338) (13.4279, 1.3445) (13.4326, 1.3478) knots 0 0 0 0 0 0 0.01428571 0.02857143 0.04285714 0.05714286 0.07142857 0.08571429 0.1 0.11428571 0.12857143 0.14285714 0.15714286 0.17142857 0.18571429 0.2 0.21428571 0.22857143 0.24285714 0.25714286 0.27142857 0.28571429 0.3 0.31428571 0.32857143 0.34285714 0.35714286 0.37142857 0.38571429 0.4 0.41428571 0.42857143 0.44285714 0.45714286 0.47142857 0.48571429 0.5 0.51428571 0.52857143 0.54285714 0.55714286 0.57142857 0.58571429 0.6 0.61428571 0.62857143 0.64285714 0.65714286 0.67142857 0.68571429 0.7 0.71428571 0.72857143 0.74285714 0.75714286 0.77142857 0.78571429 0.8 0.81428571 0.82857143 0.84285714 0.85714286 0.87142857 0.88571429 0.9 0.91428571 0.92857143 0.94285714 0.95714286 0.97142857 0.98571429 1 1 1 1 1 1
  arc A54 (13.4326, 1.3478) -> (13.3457, 2.0351) centre (0, 0) ccw
  spline S27 degree 5 poles (13.3457, 2.0351) (13.3404, 2.0371) (13.3298, 2.0411) (13.3139, 2.0471) (13.2927, 2.055) (13.2662, 2.0648) (13.2397, 2.0745) (13.2132, 2.084) (13.1867, 2.0934) (13.1602, 2.1026) (13.1337, 2.1118) (13.1072, 2.1207) (13.0806, 2.1296) (13.0541, 2.1383) (13.0276, 2.1469) (13.001, 2.1554) (12.9745, 2.1637) (12.948, 2.1719) (12.9214, 2.1799) (12.8949, 2.1879) (12.8684, 2.1956) (12.8418, 2.2033) (12.8153, 2.2107) (12.7888, 2.2181) (12.7623, 2.2253) (12.7357, 2.2324) (12.7092, 2.2393) (12.6827, 2.2461) (12.6562, 2.2527) (12.6297, 2.2592) (12.6032, 2.2655) (12.5767, 2.2717) (12.5502, 2.2777) (12.5237, 2.2835) (12.4973, 2.2893) (12.4708, 2.2948) (12.4444, 2.3002) (12.4179, 2.3055) (12.3915, 2.3105) (12.3651, 2.3155) (12.3387, 2.3202) (12.3123, 2.3248) (12.2859, 2.3292) (12.2595, 2.3335) (12.2332, 2.3375) (12.2068, 2.3414) (12.1805, 2.3451) (12.1542, 2.3487) (12.1279, 2.352) (12.1016, 2.3552) (12.0754, 2.3582) (12.0491, 2.361) (12.0229, 2.3636) (11.9968, 2.3659) (11.9706, 2.3681) (11.9445, 2.37) (11.9184, 2.3718) (11.8923, 2.3733) (11.8662, 2.3747) (11.8402, 2.3759) (11.8142, 2.3767) (11.7883, 2.3773) (11.7624, 2.3775) (11.7365, 2.3773) (11.7107, 2.3769) (11.6849, 2.3763) (11.6592, 2.3755) (11.6335, 2.3745) (11.6078, 2.3733) (11.5822, 2.3717) (11.5568, 2.3694) (11.5365, 2.3667) (11.5214, 2.3642) (11.5114, 2.3623) (11.5064, 2.3612) knots -1 -1 -1 -1 -1 -1 -0.98571429 -0.97142857 -0.95714286 -0.94285714 -0.92857143 -0.91428571 -0.9 -0.88571429 -0.87142857 -0.85714286 -0.84285714 -0.82857143 -0.81428571 -0.8 -0.78571429 -0.77142857 -0.75714286 -0.74285714 -0.72857143 -0.71428571 -0.7 -0.68571429 -0.67142857 -0.65714286 -0.64285714 -0.62857143 -0.61428571 -0.6 -0.58571429 -0.57142857 -0.55714286 -0.54285714 -0.52857143 -0.51428571 -0.5 -0.48571429 -0.47142857 -0.45714286 -0.44285714 -0.42857143 -0.41428571 -0.4 -0.38571429 -0.37142857 -0.35714286 -0.34285714 -0.32857143 -0.31428571 -0.3 -0.28571429 -0.27142857 -0.25714286 -0.24285714 -0.22857143 -0.21428571 -0.2 -0.18571429 -0.17142857 -0.15714286 -0.14285714 -0.12857143 -0.11428571 -0.1 -0.08571429 -0.07142857 -0.05714286 -0.04285714 -0.02857143 -0.01428571 0 0 0 0 0 0